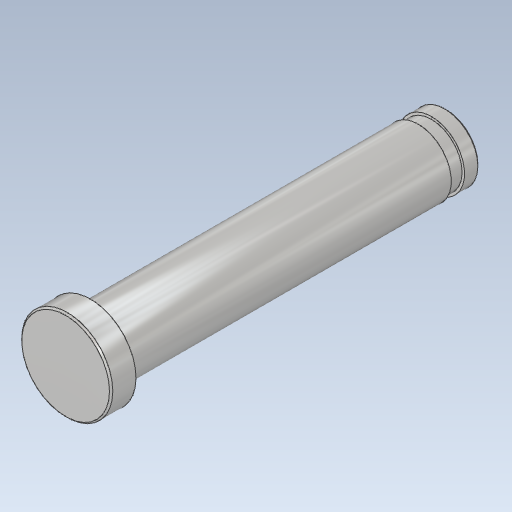
# Autodesk Inventor part: roller pin
Saved by Autodesk Inventor 2020 (Build 240168000, 168)
## iProperties
Created: 2018-11-16
Part Number: roller pin
Material: Aluminum 3003-H14
Document SubType Name: Modeling
Designer: LillaHunden
Density: 2.73809 g/cm^3
Appearance: Aluminum - Polished
Mass: 0.83297 g
Surface Area: 3.44712 cm^2
Volume: 0.304216 cm^3
Author: LillaHunden
Autodesk Inventor part; units mm, degrees
ref_plane "YZ Plane" through (0, 0, 0) normal (1, 0, 0) x (0, 1, 0)
ref_plane "XZ Plane" through (0, 0, 0) normal (0, 1, 0) x (-1, 0, 0)
sketch "Sketch1" plane through (0, 0, 0) normal (0, 0, 1) x (1, 0, 0)
  circle A0 centre (0, 0) radius 2
  dimension "d0" = 4
  constraints: 1 centre point, 1 coincident
  measures "d0" diameter of A0
extrude "Extrusion1" add sketch "Sketch1" along normal blind 21.5
sketch "Sketch2" plane through (0, 0, 21.5) normal (0, 0, 1) x (1, 0, 0)
  circle A0 centre (0, 0) radius 2.75
  dimension "d3" = 5.5
  constraints: 1 centre point, 1 coincident
  measures "d3" diameter of A0
extrude "Extrusion2" add sketch "Sketch2" along normal blind 1.5
ref_plane "Work Plane1" through (0, 0, 1.3) normal (0, 0, -1) x (-1, 0, 0)
sketch "Sketch3" plane through (0, 0, 1.3) normal (0, 0, -1) x (-1, 0, 0)
  circle A0 centre (0, 0) radius 2 projected
  circle A1 centre (0, 0) radius 1.85
  dimension "d7" = 3.7
  constraints: 1 centre point, 1 coincident
  measures "d7" diameter of A1
extrude "Extrusion3" cut sketch "Sketch3" along normal mid plane 0.8
chamfer "Chamfer1" distance 0.1 angle 45 2 edges at (-2, 0, 0) (-2.75, 0, 23)
body "Solid1"
